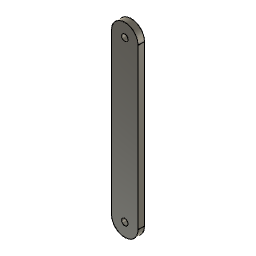
Rocker_B v2 (Autodesk Fusion 360 design; units mm, degrees)
Autodesk Fusion 360 part; units mm, degrees
sketch "Sketch1" plane through (0, 0, 0) normal (0, 1, 0) x (1, 0, 0)
  circle A0 centre (0, 96.75) radius 3
  arc A1 (12.5, 96.75) -> (-12.5, 96.75) centre (0, 96.75) ccw
  line L0 (12.5, 96.75) -> (12.5, -53.25)
  arc A2 (-12.5, -53.25) -> (12.5, -53.25) centre (0, -53.25) ccw
  line L1 (-12.5, -53.25) -> (-12.5, 96.75)
  circle A3 centre (0, -53.25) radius 3
  point P0 (-35.6168, 0)
  constraint parallel L0 L1
  constraint concentric A2 A3
extrude "Extrude1" add sketch "Sketch1" along normal blind 6
